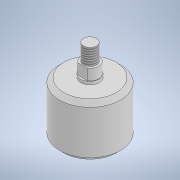
# Autodesk Inventor part: Unmodified Motor
Saved by Autodesk Inventor 2022 (Build 260153000, 153)
## iProperties
Created: 2022-08-09
Part Number: Unmodified Motor
Material: Generic
Document SubType Name: Modeling
Designer: Nick
Density: 1 g/cm^3
Appearance: Default
Author: Nick
Autodesk Inventor part; units mm, degrees
ref_plane "YZ Plane" through (0, 0, 0) normal (1, 0, 0) x (0, 1, 0)
ref_plane "XZ Plane" through (0, 0, 0) normal (0, 1, 0) x (-1, 0, 0)
ref_plane "XY Plane" through (0, 0, 0) normal (0, 0, 1) x (1, 0, 0)
sketch "Sketch1" plane through (0, 0, 0) normal (0, 0, 1) x (1, 0, 0)
  line L0 (0, 0) -> (14, 0)
  line L1 (14, 0) -> (14, 24)
  line L2 (14, 24) -> (4.25, 24)
  line L3 (4.25, 24) -> (4.25, 25.4397)
  line L4 (4.25, 25.4397) -> (4, 25.4397)
  line L5 (3, 38) -> (0, 38)
  line L6 (0, 38) -> (0, 0)
  line L7 (4, 25.4397) -> (4, 30.4397)
  line L8 (4, 30.4397) -> (3, 30.4397)
  line L9 (3, 30.4397) -> (3, 38)
  dimension "d0" = 28
  dimension "d1" = 24
  dimension "d2" = 5
  dimension "d3" = 8
  dimension "d4" = 6
  dimension "d5" = 8.5
  dimension "d6" = 38
  constraints: 20 end point, 7 perpendicular, 2 vertical, 1 horizontal
  measures "d0" diameter of L1 L6
  measures "d1" distance of L0.end L1.end
  measures "d2" distance of L4.end L7.end
  measures "d3" diameter of L7 L6
  measures "d4" diameter of L9 L6
  measures "d5" diameter of L3 L6
  measures "d6" distance of L5.end L0.start
revolve "Revolution1" add sketch "Sketch1" angle 360 about axis through (0, 38, 0) along (0, -1, 0)
chamfer "Chamfer1" distance 2 angle 45 2 edges at (-14, 0, 0) (-14, 24, 0)
thread "Thread1" size "M6x1" class "6g" standard "ANSI Metric M Profile" full length
sketch "Sketch2" plane through (0, 30.4397, 0) normal (0, 1, 0) x (1, 0, 0)
  line L0 (-2.1626, 3.365) -> (2.1626, 3.365)
  line L1 (2.1626, 3.365) -> (2.1626, -3.365)
  line L2 (2.1626, -3.365) -> (-2.1626, -3.365)
  line L3 (-2.1626, -3.365) -> (-2.1626, 3.365)
  circle A0 centre (0, 0) radius 3 projected
  circle A1 centre (0, 0) radius 4 projected
  point P0 (2.1626, 0)
  dimension "d13" = 6.73
  constraints: 8 end point, 2 parallel, 2 point on circle, 1 horizontal, 1 horizontal alignment, 1 midpoint, 1 perpendicular
  measures "d13" distance of L2.end L0.start
extrude "Extrusion1" cut sketch "Sketch2" against normal blind 5 contours A1 L0 | L2 A1
sketch "Sketch4" plane through (0, 0, 0) normal (0, -1, 0) x (1, 0, 0)
  circle A0 centre (6.7175, 6.7175) radius 1.5
  circle A1 centre (-6.7175, -6.7175) radius 1.5
  circle A2 centre (-5.6569, 5.6569) radius 1.5
  circle A3 centre (5.6569, -5.6569) radius 1.5
  line L0 (-6.7175, -6.7175) -> (6.7175, 6.7175) construction
  line L1 (-5.6569, 5.6569) -> (5.6569, -5.6569) construction
  line L2 (0, 0) -> (0, 11.5514) construction
  point P0 (0, 0)
  dimension "d20" = 3
  dimension "d21" = 19
  dimension "d22" = 16
  dimension "d23" = 45
  constraints: 6 end point, 4 centre point, 3 equal radius, 2 midpoint, 1 coincident, 1 perpendicular, 1 vertical
  measures "d20" diameter of A0
  measures "d21" distance of L0.start L0.end
  measures "d22" distance of L1.start L1.end
  measures "d23" angle of L2 L0
extrude "Extrusion3" cut sketch "Sketch4" against normal blind 5
body "Solid1"
